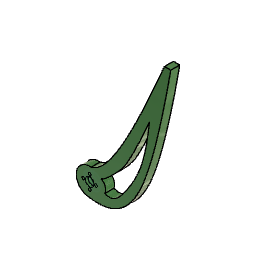
tibia v6 (Autodesk Fusion 360 design; units mm, degrees)
Autodesk Fusion 360 part; units mm, degrees
note: some values were not read from the file. Set by a fixed rule: which sketch regions a step uses.
sketch "Sketch1" plane through (0, 0, 0) normal (0, 1, 0) x (1, 0, 0)
  spline S0 degree 5 poles (-31.9133, 120.4818) (-30.7347, 120.1695) (-28.3316, 119.2929) (-24.5895, 117.2227) (-19.3204, 112.926) (-12.2476, 104.8833) (-4.6766, 94.1039) (3.3656, 80.736) (11.829, 65.0534) (20.6597, 47.3537) (29.8087, 27.9049) (37.3534, 11.1071) (43.1291, -2.1349) (47.0308, -11.2443) (48.9944, -15.8693) knots 0 0 0 0 0 0 0.1 0.2 0.3 0.4 0.5 0.6 0.7 0.8 0.9 1 1 1 1 1 1
  line L0 (56.5542, -17.0293) -> (49.487, -17.0293)
  line L1 (56.5542, -17.0293) -> (56.5542, -17.0293)
  line L2 (48.9944, -15.8693) -> (49.487, -17.0293)
  arc A0 (-34.1609, 150.3869) -> (-31.9133, 120.4818) centre (-33.4343, 135.4045) ccw
  line L3 (-34.0865, 150.3991) -> (-34.2189, 150.384)
  spline S1 degree 5 poles (-34.0865, 150.3991) (-32.2844, 150.6951) (-28.0745, 151.2424) (-21.6837, 151.5239) (-13.5056, 150.6434) (-4.1109, 147.3042) (4.7117, 141.2529) (12.4545, 132.7815) (19.2137, 122.1492) (25.1233, 109.7105) (30.334, 95.8604) (34.9946, 80.9859) (39.2349, 65.4171) (43.1506, 49.3883) (46.8097, 33.0578) (50.2562, 16.522) (52.8634, 3.1694) (54.7395, -6.9063) (55.9551, -13.6505) (56.5542, -17.0293) knots 0.018147 0.018147 0.018147 0.018147 0.018147 0.018147 0.066667 0.133333 0.2 0.266667 0.333333 0.4 0.466667 0.533333 0.6 0.666667 0.733333 0.8 0.866667 0.933333 1 1 1 1 1 1
  line L4 (-58.9956, 146.3085) -> (-9.1774, 154.4898)
  point P0 (4.2151, 140.8467)
  point P1 (34.3836, 82.5209)
  point P2 (-10.9246, 102.6332)
  dimension "d2" = 30
  constraint coincident S0.start A0
  constraint horizontal L0
  constraint vertical L1
  constraint coincident S0 A0.end
  constraint coincident A0 L3.end
  constraint midpoint L3.start L4
  measures "d2" diameter of A0
extrude "Extrude1" add sketch "Sketch1" along normal blind 15
sketch "Sketch2" plane through (0, 15, 0) normal (0, 1, 0) x (-1, 0, 0)
  arc A0 (34.2189, -150.384) -> (31.9133, -120.4818) centre (33.4343, -135.4045) ccw
  spline S0 degree 5 poles (31.9133, -120.4818) (30.7347, -120.1695) (28.3316, -119.2929) (24.5895, -117.2227) (19.3204, -112.926) (12.2476, -104.8833) (4.6766, -94.1039) (-3.3656, -80.736) (-11.829, -65.0534) (-20.6597, -47.3537) (-29.8087, -27.9049) (-37.3534, -11.1071) (-43.1291, 2.1349) (-47.0308, 11.2443) (-48.9944, 15.8693) knots 0 0 0 0 0 0 0.1 0.2 0.3 0.4 0.5 0.6 0.7 0.8 0.9 1 1 1 1 1 1
  line L0 (-48.9944, 15.8693) -> (-49.487, 17.0293)
  line L1 (-49.487, 17.0293) -> (-56.5542, 17.0293)
  spline S1 degree 5 poles (-56.5542, 17.0293) (-55.9551, 13.6505) (-54.7395, 6.9063) (-52.8634, -3.1694) (-50.2562, -16.522) (-46.8097, -33.0578) (-43.1506, -49.3883) (-39.2349, -65.4171) (-34.9946, -80.9859) (-30.334, -95.8604) (-25.1233, -109.7105) (-19.2137, -122.1492) (-12.4545, -132.7815) (-4.7117, -141.2529) (4.1109, -147.3042) (13.5056, -150.6434) (21.6837, -151.5239) (28.0745, -151.2424) (32.2844, -150.6951) (34.0865, -150.3991) knots -1 -1 -1 -1 -1 -1 -0.933333 -0.866667 -0.8 -0.733333 -0.666667 -0.6 -0.533333 -0.466667 -0.4 -0.333333 -0.266667 -0.2 -0.133333 -0.066667 -0.018147 -0.018147 -0.018147 -0.018147 -0.018147 -0.018147
  line L2 (34.0865, -150.3991) -> (34.2189, -150.384)
  circle A1 centre (33.4343, -135.4045) radius 15
  circle A2 centre (33.4343, -135.4045) radius 10
  dimension "d5" = 30
  dimension "d6" = 20
  constraint coincident A0.centre A1.centre
  constraint concentric A1 A2
  measures "d5" diameter of A1
  measures "d6" diameter of A2
extrude "Extrude2" cut sketch "Sketch2" against normal blind 3 contours A2
sketch "Sketch3" plane through (0, 15, 0) normal (0, 1, 0) x (-1, 0, 0)
  circle A0 centre (33.4343, -135.4045) radius 10
  arc A1 (34.2189, -150.384) -> (31.9133, -120.4818) centre (33.4343, -135.4045) ccw
  spline S0 degree 5 poles (31.9133, -120.4818) (30.7347, -120.1695) (28.3316, -119.2929) (24.5895, -117.2227) (19.3204, -112.926) (12.2476, -104.8833) (4.6766, -94.1039) (-3.3656, -80.736) (-11.829, -65.0534) (-20.6597, -47.3537) (-29.8087, -27.9049) (-37.3534, -11.1071) (-43.1291, 2.1349) (-47.0308, 11.2443) (-48.9944, 15.8693) knots 0 0 0 0 0 0 0.1 0.2 0.3 0.4 0.5 0.6 0.7 0.8 0.9 1 1 1 1 1 1
  line L0 (-48.9944, 15.8693) -> (-49.487, 17.0293)
  line L1 (-49.487, 17.0293) -> (-56.5542, 17.0293)
  spline S1 degree 5 poles (-56.5542, 17.0293) (-55.9551, 13.6505) (-54.7395, 6.9063) (-52.8634, -3.1694) (-50.2562, -16.522) (-46.8097, -33.0578) (-43.1506, -49.3883) (-39.2349, -65.4171) (-34.9946, -80.9859) (-30.334, -95.8604) (-25.1233, -109.7105) (-19.2137, -122.1492) (-12.4545, -132.7815) (-4.7117, -141.2529) (4.1109, -147.3042) (13.5056, -150.6434) (21.6837, -151.5239) (28.0745, -151.2424) (32.2844, -150.6951) (34.0865, -150.3991) knots -1 -1 -1 -1 -1 -1 -0.933333 -0.866667 -0.8 -0.733333 -0.666667 -0.6 -0.533333 -0.466667 -0.4 -0.333333 -0.266667 -0.2 -0.133333 -0.066667 -0.018147 -0.018147 -0.018147 -0.018147 -0.018147 -0.018147
  line L2 (34.0865, -150.3991) -> (34.2189, -150.384)
  spline S2 degree 5 poles (20.7681, -125.9637) (20.5132, -126.1) (20.0185, -126.382) (19.322, -126.8334) (18.4858, -127.4929) (17.605, -128.4197) (16.9022, -129.4566) (16.3906, -130.6107) (16.0743, -131.8817) (15.9427, -133.2614) (15.9806, -134.74) (16.1347, -135.9947) (16.3153, -136.9734) (16.4642, -137.6424) (16.5458, -137.981) knots 0 0 0 0 0 0 0.1 0.2 0.3 0.4 0.5 0.6 0.7 0.8 0.9 1 1 1 1 1 1
  spline S3 degree 5 poles (16.5458, -137.981) (15.8961, -138.3254) (14.6002, -138.9051) (12.6668, -139.4475) (10.1096, -139.5136) (6.9484, -138.5131) (3.8235, -136.4908) (0.736, -133.5981) (-2.3114, -130.0435) (-5.3132, -126.0431) (-8.2596, -121.7828) (-11.1349, -117.365) (-13.9177, -112.8002) (-16.5839, -108.0404) (-19.1096, -103.0007) (-21.4729, -97.5841) (-23.6579, -91.7079) (-25.6557, -85.3214) (-27.463, -78.3959) (-29.0795, -70.9199) (-30.5076, -62.8922) (-31.5014, -56.0326) (-32.1643, -50.6447) (-32.5698, -46.9451) (-32.7634, -45.0684) knots 0 0 0 0 0 0 0.05 0.1 0.15 0.2 0.25 0.3 0.35 0.4 0.45 0.5 0.55 0.6 0.65 0.7 0.75 0.8 0.85 0.9 0.95 1 1 1 1 1 1
  spline S4 degree 5 poles (20.7681, -125.9637) (20.2796, -125.8348) (19.2342, -125.4491) (17.4617, -124.4883) (14.6775, -122.4227) (10.6128, -118.7037) (6.1821, -114.1481) (2.1641, -109.9253) (-1.219, -106.2119) (-4.2789, -102.3084) (-7.4329, -97.4121) (-10.937, -91.1468) (-14.5785, -84.1289) (-18.285, -76.6259) (-21.9828, -68.8763) (-25.641, -60.9976) (-28.5209, -54.6462) (-30.6529, -49.8642) (-32.062, -46.6683) (-32.7634, -45.0684) knots 0 0 0 0 0 0 0.066667 0.133333 0.2 0.266667 0.333333 0.4 0.466667 0.533333 0.6 0.666667 0.733333 0.8 0.866667 0.933333 1 1 1 1 1 1
  line L3 (-3.6517, -103.8458) -> (-13.5936, -86.5321)
  line L4 (15.9112, -124.1088) -> (-1.422, -106.3252)
  line L5 (17.0248, -129.1186) -> (16.0667, -131.5781)
  point P0 (16.5458, -130.3484)
  point P1 (6.4096, -137.981)
  point P2 (-6.7871, -123.8744)
  point P3 (-20.8755, -98.8185)
  point P4 (7.2446, -115.217)
  point P5 (-8.6226, -95.1889)
  constraint midpoint P5 L3
  constraint midpoint P4 L4
  constraint midpoint P0 L5
extrude "Extrude3" cut sketch "Sketch3" against normal blind 15 contours S2 S3 S4
sketch "Sketch4" plane through (0, 0, 0) normal (0, -1, 0) x (1, 0, 0)
  spline S0 degree 5 poles (-20.7681, -125.9637) (-20.2796, -125.8348) (-19.2342, -125.4491) (-17.4617, -124.4883) (-14.6775, -122.4227) (-10.6128, -118.7037) (-6.1821, -114.1481) (-2.1641, -109.9253) (1.219, -106.2119) (4.2789, -102.3084) (7.4329, -97.4121) (10.937, -91.1468) (14.5785, -84.1289) (18.285, -76.6259) (21.9828, -68.8763) (25.641, -60.9976) (28.5209, -54.6462) (30.6529, -49.8642) (32.062, -46.6683) (32.7634, -45.0684) knots 0 0 0 0 0 0 0.066667 0.133333 0.2 0.266667 0.333333 0.4 0.466667 0.533333 0.6 0.666667 0.733333 0.8 0.866667 0.933333 1 1 1 1 1 1
  spline S1 degree 5 poles (32.7634, -45.0684) (32.5698, -46.9451) (32.1643, -50.6447) (31.5014, -56.0326) (30.5076, -62.8922) (29.0795, -70.9199) (27.463, -78.3959) (25.6557, -85.3214) (23.6579, -91.7079) (21.4729, -97.5841) (19.1096, -103.0007) (16.5839, -108.0404) (13.9177, -112.8002) (11.1349, -117.365) (8.2596, -121.7828) (5.3132, -126.0431) (2.3114, -130.0435) (-0.736, -133.5981) (-3.8235, -136.4908) (-6.9484, -138.5131) (-10.1096, -139.5136) (-12.6668, -139.4475) (-14.6002, -138.9051) (-15.8961, -138.3254) (-16.5458, -137.981) knots -1 -1 -1 -1 -1 -1 -0.95 -0.9 -0.85 -0.8 -0.75 -0.7 -0.65 -0.6 -0.55 -0.5 -0.45 -0.4 -0.35 -0.3 -0.25 -0.2 -0.15 -0.1 -0.05 0 0 0 0 0 0
  spline S2 degree 5 poles (-16.5458, -137.981) (-16.4642, -137.6424) (-16.3153, -136.9734) (-16.1347, -135.9947) (-15.9806, -134.74) (-15.9427, -133.2614) (-16.0743, -131.8817) (-16.3906, -130.6107) (-16.9022, -129.4566) (-17.605, -128.4197) (-18.4858, -127.4929) (-19.322, -126.8334) (-20.0185, -126.382) (-20.5132, -126.1) (-20.7681, -125.9637) knots -1 -1 -1 -1 -1 -1 -0.9 -0.8 -0.7 -0.6 -0.5 -0.4 -0.3 -0.2 -0.1 0 0 0 0 0 0
  arc A0 (-31.9133, -120.4818) -> (-34.2189, -150.384) centre (-33.4343, -135.4045) ccw
  line L0 (-34.2189, -150.384) -> (-34.0865, -150.3991)
  spline S3 degree 5 poles (-34.0865, -150.3991) (-32.2844, -150.6951) (-28.0745, -151.2424) (-21.6837, -151.5239) (-13.5056, -150.6434) (-4.1109, -147.3042) (4.7117, -141.2529) (12.4545, -132.7815) (19.2137, -122.1492) (25.1233, -109.7105) (30.334, -95.8604) (34.9946, -80.9859) (39.2349, -65.4171) (43.1506, -49.3883) (46.8097, -33.0578) (50.2562, -16.522) (52.8634, -3.1694) (54.7395, 6.9063) (55.9551, 13.6505) (56.5542, 17.0293) knots 0.018147 0.018147 0.018147 0.018147 0.018147 0.018147 0.066667 0.133333 0.2 0.266667 0.333333 0.4 0.466667 0.533333 0.6 0.666667 0.733333 0.8 0.866667 0.933333 1 1 1 1 1 1
  line L1 (56.5542, 17.0293) -> (49.487, 17.0293)
  line L2 (49.487, 17.0293) -> (48.9944, 15.8693)
  spline S4 degree 5 poles (-31.9133, -120.4818) (-30.7347, -120.1695) (-28.3316, -119.2929) (-24.5895, -117.2227) (-19.3204, -112.926) (-12.2476, -104.8833) (-4.6766, -94.1039) (3.3656, -80.736) (11.829, -65.0534) (20.6597, -47.3537) (29.8087, -27.9049) (37.3534, -11.1071) (43.1291, 2.1349) (47.0308, 11.2443) (48.9944, 15.8693) knots 0 0 0 0 0 0 0.1 0.2 0.3 0.4 0.5 0.6 0.7 0.8 0.9 1 1 1 1 1 1
  circle A1 centre (-33.4343, -135.4045) radius 15
  circle A2 centre (-33.4343, -135.4045) radius 10
  dimension "d11" = 30
  dimension "d12" = 20
  constraint coincident A0.centre A1.centre
  constraint concentric A0 A2
  measures "d11" diameter of A1
  measures "d12" diameter of A2
extrude "Extrude4" cut sketch "Sketch4" against normal blind 3 contours A2
extrude "Extrude5" cut 1 faces at (32.4368, 0, -28.8776) along direction (0, 1, 0) blind 5
sketch "Sketch5" plane through (0, 12, 0) normal (0, 1, 0) x (-1, 0, 0)
  circle A0 centre (33.4343, -135.4045) radius 10
  circle A1 centre (33.4343, -135.4045) radius 10
  line L0 (33.4343, -135.4045) -> (40.4343, -135.4045)
  circle A2 centre (40.4343, -135.4045) radius 1.5
  circle A3 centre (33.4343, -135.4045) radius 2.5
  line L1 (33.4343, -135.4045) -> (33.4343, -135)
  line L2 (33.4343, -135) -> (33.4343, -128)
  circle A4 centre (33.4343, -128) radius 1.5
  circle A5 centre (33.4343, -142.809) radius 1.5
  circle A6 centre (26.4343, -135.4045) radius 1.5
  dimension "d17" = 7
  dimension "d18" = 3
  dimension "d19" = 5
  dimension "d20" = 7
  dimension "d21" = 3
  constraint concentric A0 A1
  constraint coincident A0.centre A1.centre
  constraint horizontal L0
  constraint coincident L0.end A2.centre
  constraint concentric A1 A3
  constraint perpendicular L0 L1
  constraint perpendicular L0 L2
  constraint coincident L2.end A4.centre
  constraint symmetric L0 A4 A5
  constraint symmetric A2 L2 A6
  measures "d17" distance of A0.centre L0.end
  measures "d18" diameter of A2
  measures "d19" diameter of A3
  measures "d20" distance of L1.end L2.end
  measures "d21" diameter of A4
extrude "Extrude6" cut sketch "Sketch5" against normal blind 10 contours L0 A3 L1 L2 | L0 A3 L1 L2 | A2 | A4 | A5 | A6
extrude "Extrude7" cut 1 faces at (-28.4944, 3, -130.5177) along direction (0, 1, 0) blind 2
extrude "Extrude8" cut 1 faces at (-38.3743, 12, -130.5177) along direction (0, -1, 0) blind 3
sketch "Sketch6" plane through (0, 5, 0) normal (0, -1, 0) x (1, 0, 0)
  circle A0 centre (-33.4343, -142.809) radius 1.5
  circle A1 centre (-26.4343, -135.4045) radius 1.5
  circle A2 centre (-40.4343, -135.4045) radius 1.5
  circle A3 centre (-33.4343, -128) radius 1.5
  circle A4 centre (-33.4343, -135.4045) radius 2.5
  spline S0 degree 3 poles (32.7634, -45.0684) (27.6878, -56.6459) (21.7944, -69.521) (8.2028, -96.9385) (4.5984, -102.0744) (-1.9434, -109.8084) (-8.3618, -116.465) (-13.6185, -121.4376) (-16.0409, -123.5269) (-18.9925, -125.2819) (-19.8904, -125.7321) (-20.7681, -125.9637) knots -4.240539 -4.240539 -4.240539 -4.240539 -3.375006 -3.375006 -2.08069 -2.08069 -1.032044 -1.032044 -0.272306 -0.272306 0 0 0 0
  spline S1 degree 3 poles (-16.5458, -137.981) (-15.5835, -138.4911) (-14.5663, -138.8891) (-12.5052, -139.3338) (-11.5014, -139.3943) (-9.0449, -139.1389) (-7.6874, -138.6641) (-4.2059, -136.8029) (-2.0085, -134.8859) (5.1366, -126.8808) (11.6945, -116.8753) (22.3963, -97.2985) (29.11, -80.4832) (32.7634, -45.0684) knots -24.656813 -24.656813 -24.656813 -24.656813 -23.305659 -23.305659 -22.042082 -22.042082 -20.244188 -20.244188 -17.147446 -17.147446 -10.68083 -10.68083 0 0 0 0
  spline S2 degree 3 poles (-20.7681, -125.9637) (-19.9485, -126.4018) (-19.1626, -126.9309) (-17.8409, -128.152) (-17.3001, -128.8238) (-16.4524, -130.4209) (-16.1475, -131.3902) (-15.8389, -134.5443) (-16.2031, -136.5586) (-16.5458, -137.981) knots -1.222468 -1.222468 -1.222468 -1.222468 -0.955706 -0.955706 -0.706259 -0.706259 -0.438917 -0.438917 0 0 0 0
  arc A5 (-31.9133, -120.4818) -> (-34.2189, -150.384) centre (-33.4343, -135.4045) ccw
  line L0 (-34.2189, -150.384) -> (-34.0865, -150.3991)
  spline S3 degree 3 poles (56.5542, 17.0293) (52.9419, -3.3448) (48.6575, -25.0592) (39.2886, -65.927) (33.9271, -86.0394) (23.4961, -113.6189) (18.7964, -123.1311) (9.8702, -135.5392) (5.7548, -140.0031) (-3.6784, -146.7116) (-8.6082, -148.9239) (-20.6088, -151.6174) (-27.4246, -151.4932) (-34.0865, -150.3991) knots -15.964393 -15.964393 -15.964393 -15.964393 -12.209093 -12.209093 -8.270793 -8.270793 -5.489128 -5.489128 -3.684114 -3.684114 -2.025345 -2.025345 0 0 0 0
  line L1 (56.5542, 17.0293) -> (49.487, 17.0293)
  line L2 (49.487, 17.0293) -> (48.9944, 15.8693)
  spline S4 degree 3 poles (-31.9133, -120.4818) (-29.1359, -119.7457) (-26.5053, -118.2503) (-21.111, -114.2973) (-18.235, -111.4275) (-9.1962, -101.1359) (-2.722, -91.0449) (17.9098, -54.7727) (34.4233, -18.4507) (48.9944, 15.8693) knots -19.22208 -19.22208 -19.22208 -19.22208 -17.829954 -17.829954 -15.982961 -15.982961 -11.185534 -11.185534 0 0 0 0
  circle A6 centre (-33.4343, -135.4045) radius 4
  circle A7 centre (-33.4343, -128) radius 2
  circle A8 centre (-26.4343, -135.4045) radius 2
  circle A9 centre (-33.4343, -142.809) radius 2
  circle A10 centre (-40.4343, -135.4045) radius 2
  dimension "d28" = 8
  dimension "d29" = 4
  dimension "d30" = 4
  dimension "d31" = 4
  dimension "d32" = 4
  constraint concentric A4 A6
  constraint concentric A3 A7
  constraint concentric A1 A8
  constraint concentric A0 A9
  constraint concentric A2 A10
  measures "d28" diameter of A6
  measures "d29" diameter of A7
  measures "d30" diameter of A8
  measures "d31" diameter of A9
  measures "d32" diameter of A10
extrude "Extrude9" cut sketch "Sketch6" against normal blind 19 contours A6 | A7 | A8 | A9 | A10
extrude "Extrude10" cut 1 faces at (-38.945, 9, -139.1992) along direction (0, -1, 0) blind 1
sketch "Sketch7" plane through (0, 5, 0) normal (0, -1, 0) x (1, 0, 0)
  circle A0 centre (-40.4343, -135.4045) radius 2
  circle A1 centre (-33.4343, -128) radius 2
  circle A2 centre (-33.4343, -142.809) radius 2
  circle A3 centre (-33.4343, -135.4045) radius 4
  circle A4 centre (-26.4343, -135.4045) radius 2
  spline S0 degree 3 poles (32.7634, -45.0684) (27.6878, -56.6459) (21.7944, -69.521) (8.2028, -96.9385) (4.5984, -102.0744) (-1.9434, -109.8084) (-8.3618, -116.465) (-13.6185, -121.4376) (-16.0409, -123.5269) (-18.9925, -125.2819) (-19.8904, -125.7321) (-20.7681, -125.9637) knots -4.240539 -4.240539 -4.240539 -4.240539 -3.375006 -3.375006 -2.08069 -2.08069 -1.032044 -1.032044 -0.272306 -0.272306 0 0 0 0
  spline S1 degree 3 poles (-16.5458, -137.981) (-15.5835, -138.4911) (-14.5663, -138.8891) (-12.5052, -139.3338) (-11.5014, -139.3943) (-9.0449, -139.1389) (-7.6874, -138.6641) (-4.2059, -136.8029) (-2.0085, -134.8859) (5.1366, -126.8808) (11.6945, -116.8753) (22.3963, -97.2985) (29.11, -80.4832) (32.7634, -45.0684) knots -24.656813 -24.656813 -24.656813 -24.656813 -23.305659 -23.305659 -22.042082 -22.042082 -20.244188 -20.244188 -17.147446 -17.147446 -10.68083 -10.68083 0 0 0 0
  spline S2 degree 3 poles (-20.7681, -125.9637) (-19.9485, -126.4018) (-19.1626, -126.9309) (-17.8409, -128.152) (-17.3001, -128.8238) (-16.4524, -130.4209) (-16.1475, -131.3902) (-15.8389, -134.5443) (-16.2031, -136.5586) (-16.5458, -137.981) knots -1.222468 -1.222468 -1.222468 -1.222468 -0.955706 -0.955706 -0.706259 -0.706259 -0.438917 -0.438917 0 0 0 0
  arc A5 (-31.9133, -120.4818) -> (-34.2189, -150.384) centre (-33.4343, -135.4045) ccw
  line L0 (-34.2189, -150.384) -> (-34.0865, -150.3991)
  spline S3 degree 3 poles (56.5542, 17.0293) (52.9419, -3.3448) (48.6575, -25.0592) (39.2886, -65.927) (33.9271, -86.0394) (23.4961, -113.6189) (18.7964, -123.1311) (9.8702, -135.5392) (5.7548, -140.0031) (-3.6784, -146.7116) (-8.6082, -148.9239) (-20.6088, -151.6174) (-27.4246, -151.4932) (-34.0865, -150.3991) knots -15.964393 -15.964393 -15.964393 -15.964393 -12.209093 -12.209093 -8.270793 -8.270793 -5.489128 -5.489128 -3.684114 -3.684114 -2.025345 -2.025345 0 0 0 0
  line L1 (56.5542, 17.0293) -> (49.487, 17.0293)
  line L2 (49.487, 17.0293) -> (48.9944, 15.8693)
  spline S4 degree 3 poles (-31.9133, -120.4818) (-29.1359, -119.7457) (-26.5053, -118.2503) (-21.111, -114.2973) (-18.235, -111.4275) (-9.1962, -101.1359) (-2.722, -91.0449) (17.9098, -54.7727) (34.4233, -18.4507) (48.9944, 15.8693) knots -19.22208 -19.22208 -19.22208 -19.22208 -17.829954 -17.829954 -15.982961 -15.982961 -11.185534 -11.185534 0 0 0 0
  circle A6 centre (-33.4343, -135.4045) radius 4.75
  circle A7 centre (-33.4343, -128) radius 2
  circle A8 centre (-33.4343, -128) radius 1.5
  dimension "d37" = 9.5
  dimension "d38" = 3
  constraint concentric A3 A6
  constraint concentric A1 A7
  constraint concentric A7 A8
  measures "d37" diameter of A6
  measures "d38" diameter of A8
extrude "Extrude11" cut sketch "Sketch7" against normal blind 22 contours A6
sketch "Sketch8" plane through (0, 5, 0) normal (0, -1, 0) x (1, 0, 0)
  circle A0 centre (-33.4343, -135.4045) radius 4.75
  circle A1 centre (-40.4343, -135.4045) radius 2
  circle A2 centre (-33.4343, -128) radius 2
  circle A3 centre (-33.4343, -142.809) radius 2
  circle A4 centre (-26.4343, -135.4045) radius 2
  spline S0 degree 3 poles (32.7634, -45.0684) (27.6878, -56.6459) (21.7944, -69.521) (8.2028, -96.9385) (4.5984, -102.0744) (-1.9434, -109.8084) (-8.3618, -116.465) (-13.6185, -121.4376) (-16.0409, -123.5269) (-18.9925, -125.2819) (-19.8904, -125.7321) (-20.7681, -125.9637) knots -4.240539 -4.240539 -4.240539 -4.240539 -3.375006 -3.375006 -2.08069 -2.08069 -1.032044 -1.032044 -0.272306 -0.272306 0 0 0 0
  spline S1 degree 3 poles (-16.5458, -137.981) (-15.5835, -138.4911) (-14.5663, -138.8891) (-12.5052, -139.3338) (-11.5014, -139.3943) (-9.0449, -139.1389) (-7.6874, -138.6641) (-4.2059, -136.8029) (-2.0085, -134.8859) (5.1366, -126.8808) (11.6945, -116.8753) (22.3963, -97.2985) (29.11, -80.4832) (32.7634, -45.0684) knots -24.656813 -24.656813 -24.656813 -24.656813 -23.305659 -23.305659 -22.042082 -22.042082 -20.244188 -20.244188 -17.147446 -17.147446 -10.68083 -10.68083 0 0 0 0
  spline S2 degree 3 poles (-20.7681, -125.9637) (-19.9485, -126.4018) (-19.1626, -126.9309) (-17.8409, -128.152) (-17.3001, -128.8238) (-16.4524, -130.4209) (-16.1475, -131.3902) (-15.8389, -134.5443) (-16.2031, -136.5586) (-16.5458, -137.981) knots -1.222468 -1.222468 -1.222468 -1.222468 -0.955706 -0.955706 -0.706259 -0.706259 -0.438917 -0.438917 0 0 0 0
  arc A5 (-31.9133, -120.4818) -> (-34.2189, -150.384) centre (-33.4343, -135.4045) ccw
  line L0 (-34.2189, -150.384) -> (-34.0865, -150.3991)
  spline S3 degree 3 poles (56.5542, 17.0293) (52.9419, -3.3448) (48.6575, -25.0592) (39.2886, -65.927) (33.9271, -86.0394) (23.4961, -113.6189) (18.7964, -123.1311) (9.8702, -135.5392) (5.7548, -140.0031) (-3.6784, -146.7116) (-8.6082, -148.9239) (-20.6088, -151.6174) (-27.4246, -151.4932) (-34.0865, -150.3991) knots -15.964393 -15.964393 -15.964393 -15.964393 -12.209093 -12.209093 -8.270793 -8.270793 -5.489128 -5.489128 -3.684114 -3.684114 -2.025345 -2.025345 0 0 0 0
  line L1 (56.5542, 17.0293) -> (49.487, 17.0293)
  line L2 (49.487, 17.0293) -> (48.9944, 15.8693)
  spline S4 degree 3 poles (-31.9133, -120.4818) (-29.1359, -119.7457) (-26.5053, -118.2503) (-21.111, -114.2973) (-18.235, -111.4275) (-9.1962, -101.1359) (-2.722, -91.0449) (17.9098, -54.7727) (34.4233, -18.4507) (48.9944, 15.8693) knots -19.22208 -19.22208 -19.22208 -19.22208 -17.829954 -17.829954 -15.982961 -15.982961 -11.185534 -11.185534 0 0 0 0
  circle A6 centre (-33.4343, -128) radius 2
  circle A7 centre (-26.4343, -135.4045) radius 1.5
  circle A8 centre (-33.4343, -142.809) radius 1.5
  circle A9 centre (-40.4343, -135.4045) radius 1.5
  circle A10 centre (-33.4343, -128) radius 1.5
  dimension "d41" = 3
  dimension "d42" = 3
  dimension "d43" = 3
  dimension "d44" = 3
  constraint concentric A2 A6
  constraint concentric A4 A7
  constraint concentric A3 A8
  constraint concentric A1 A9
  constraint concentric A6 A10
  measures "d41" diameter of A7
  measures "d42" diameter of A8
  measures "d43" diameter of A9
  measures "d44" diameter of A10
extrude "Extrude12" add sketch "Sketch8" against normal blind 3 contours A1 | A2 A6 | A3 | A4
sketch "Sketch9" plane through (0, 8, 0) normal (0, 1, 0) x (-1, 0, 0)
  circle A0 centre (33.4343, -142.809) radius 1.5
  circle A1 centre (33.4343, -128) radius 1.5
  circle A2 centre (26.4343, -135.4045) radius 1.5
  circle A3 centre (40.4343, -135.4045) radius 1.5
  circle A4 centre (33.4343, -135.4045) radius 4.75
  circle A5 centre (33.4343, -135.4045) radius 10
